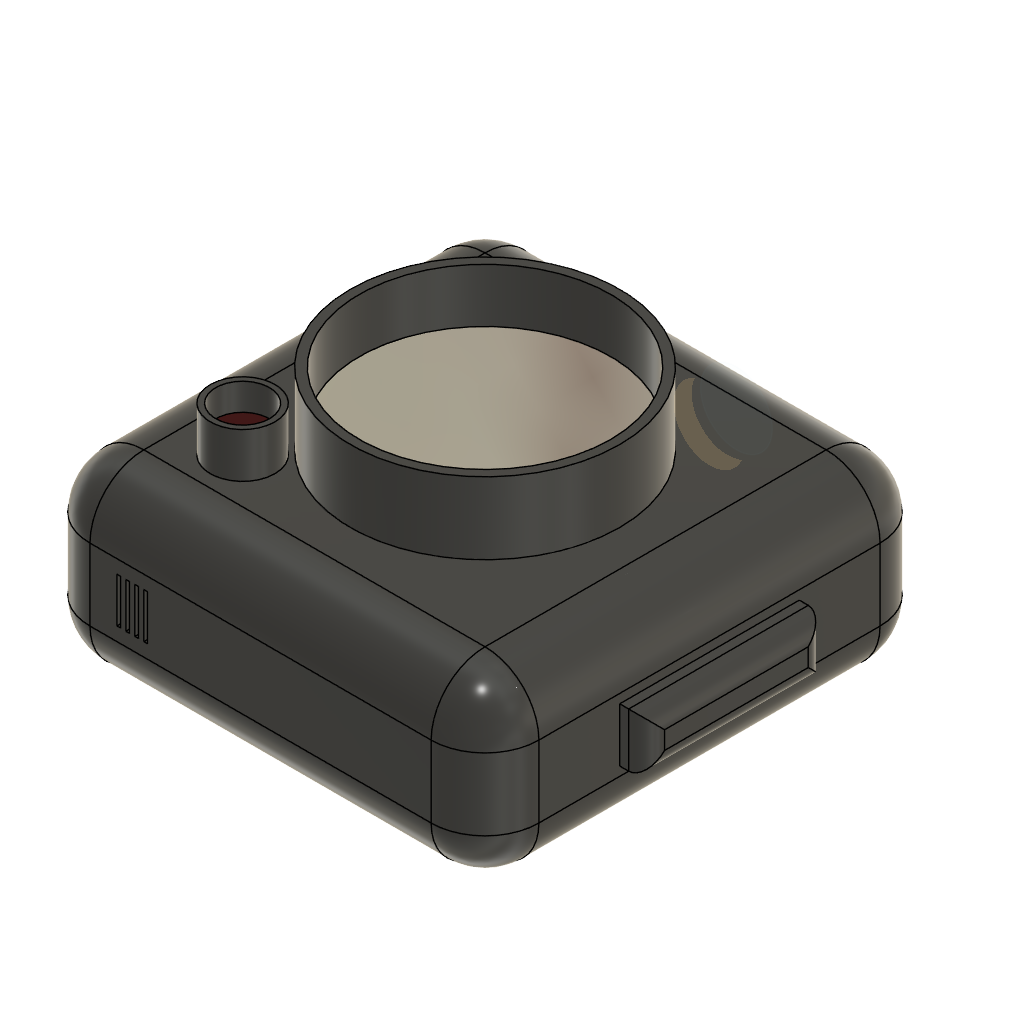
headlight_model___ (Autodesk Fusion 360 archive; units mm, degrees)
design "body"
part number: 2026-09-10-13-23-47-843
Autodesk Fusion 360 part; units mm, degrees
box "BoxPrimitive1" add length 50 width 50 height 20 placed x (0, 1, 0) y (-1, 0, 0) z (0, 0, 1) at (50, 0, 0)
fillet "Fillet1" radius 6 6 faces at (0, 33.3333, 6.6667) (33.3333, 0, 6.6667) (33.3333, 50, 6.6667) (16.6667, 16.6667, 20) (16.6667, 16.6667, 0) (50, 33.3333, 6.6667)
cylinder "CylinderPrimitive1" add diameter 30 height 5 placed x (1, 0, 0) y (0, 1, 0) z (0, 0, 1) at (25, 25, 20)
sketch "Sketch3" plane through (0, 0, 25) normal (0, 0, 1) x (-1, 0, 0)
  circle A0 centre (-25, -25) radius 15
extrude "Extrude1" add sketch "Sketch3" along normal blind 3
hole "Hole1" at (25, 25, 28) direction (0, 0, -1) diameter 28 depth 10 tip angle 180
extrude "Extrude2" add 1 faces at (28.0299, 26.6436, 18) along direction (0, 0, 1) blind 4
cylinder "CylinderPrimitive2" add diameter 7.211 height 5 placed x (1, 0, 0) y (0, 1, 0) z (0, 0, 1) at (12, 11, 20)
hole "Hole2" at (12, 11, 25) direction (0, 0, -1) diameter 6 depth 3 tip angle 180
cylinder "CylinderPrimitive3" add diameter 8 height 3 placed x (1, 0, 0) y (0, 0, -1) z (0, 1, 0) at (25, 50, 10)
sketch "Sketch6" plane through (0, 53, 0) normal (0, 1, 0) x (-1, 0, 0)
  circle A0 centre (-25, 10) radius 4
fillet "Fillet2" radius 1 1 faces at (24.6775, 53, 8.8711)
box "BoxPrimitive2" cut length 4.988 width 0.4 height -5 placed x (0, 0, 1) y (-1, 0, 0) z (0, -1, 0) at (9.4, 0, 7.5123)
box "BoxPrimitive3" cut length 4.985 width 0.4 height -5 placed x (0, 0, 1) y (-1, 0, 0) z (0, -1, 0) at (10.4, 0, 7.5)
box "BoxPrimitive4" cut length 5.005 width 0.4 height -5 placed x (0, 0, 1) y (-1, 0, 0) z (0, -1, 0) at (11.4, 0, 7.5)
box "BoxPrimitive5" cut length 5.015 width 0.4 height -5 placed x (0, 0, 1) y (-1, 0, 0) z (0, -1, 0) at (12.4, 0, 7.5)
box "BoxPrimitive6" add length 6 width 20 height 3 placed x (0, 0, -1) y (0, 1, 0) z (1, 0, 0) at (50, 15, 13)
fillet "Fillet3" radius 2 1 faces at (53, 28.3333, 11)
